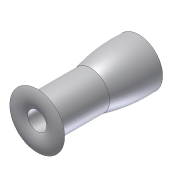
# Autodesk Inventor part: HW-00010
Saved by Autodesk Inventor 2012 (Build 160160000, 160)
## iProperties
Created: 2008-05-28
Part Number: HW-00010
Description: Pop Rivet 3/16 Dia.
Document SubType Name: Modeling
Designer: narosenberg
Density: 1 g/cm^3
Mass: 0.22468 g
Surface Area: 3.8255 cm^2
Volume: 0.22468 cm^3
Material: Default
Author: narosenberg
Autodesk Inventor part; units mm, degrees
ref_plane "YZ Plane" through (0, 0, 0) normal (1, 0, 0) x (0, 1, 0)
ref_plane "XY Plane" through (0, 0, 0) normal (0, 0, 1) x (1, 0, 0)
sketch "Sketch1" plane through (0, 0, 0) normal (0, 0, 1) x (1, 0, 0)
  circle A0 centre (-20.6161, 18.1675) radius 2.3813
  circle A1 centre (-20.6161, 18.1675) radius 1.1848
  dimension "d0" = 4.7625
  constraints: 2 centre point, 1 coincident
  measures "d0" diameter of A0
extrude "Extrusion1" add sketch "Sketch1" along normal blind 12.7
ref_plane "Work Plane1" through (-20.6161, 18.1675, 0) normal (-1, 0, 0) x (0, 0, 1)
sketch "Sketch2" plane through (-20.6161, 18.1675, 0) normal (-1, 0, 0) x (0, 0, 1)
  line L0 (0, 1.1848) -> (12.7, 1.1848) projected
  line L1 (0, -1.1848) -> (12.7, -1.1848) projected
  line L2 (12.7, 1.1848) -> (12.7, -1.1848) projected
  line L3 (12.7, 2.3813) -> (12.7, -2.3812) projected
  arc A0 (12.7, 1.1848) -> (12.7, 3.4445) centre (11.0585, 2.3147) ccw
  line L4 (12.7, 3.4445) -> (12.7, 1.1848)
  line L5 (-2.54, 0) -> (15.24, 0) projected
  constraints: 2 end point, 2 point on circle, 1 centre point, 1 collinear
revolve "Revolution1" add sketch "Sketch2" angle 360 about axis through (-20.6161, 18.1675, 0) along (0, 0, 1)
sketch "Sketch3" plane through (-20.6161, 18.1675, 0) normal (-1, 0, 0) x (0, 0, 1)
  line L0 (12.7, -3.4445) -> (12.7, -2.3812) projected
  line L1 (12.7, -2.3812) -> (0, -2.3812) projected
  line L2 (0, -2.3812) -> (0, -1.1848) projected
  line L3 (0, -1.1848) -> (12.7, -1.1848) projected
  arc A0 (12.7, -3.4445) -> (12.7, -1.1848) centre (11.0585, -2.3147) ccw projected
  line L4 (12.7, 2.3813) -> (12.7, 3.4445) projected
  arc A1 (12.7, 1.1848) -> (12.7, 3.4445) centre (11.0585, 2.3147) ccw projected
  line L5 (12.7, 1.1848) -> (0, 1.1848) projected
  line L6 (0, 1.1848) -> (0, 2.3813) projected
  line L7 (0, 2.3813) -> (12.7, 2.3813) projected
  line L8 (-2.6102, 0) -> (15.6615, 0) projected
  arc A2 (5.9963, 2.3813) -> (-0.0511, 2.9836) centre (1.0853, -16.2648) ccw
  line L9 (-0.0511, 2.9836) -> (-0.0511, 2.3813)
  line L10 (5.9963, 2.3813) -> (-0.0511, 2.3813)
  point P0 (6.35, 2.3813)
  constraints: 4 end point, 2 point on circle, 2 point on line, 1 centre point, 1 collinear, 1 midpoint, 1 perpendicular
revolve "Revolution3" add sketch "Sketch3" angle 360 about axis through (-20.6161, 18.1675, 0) along (0, 0, 1) contours L7 L10 L9 A2
body "Solid1"
